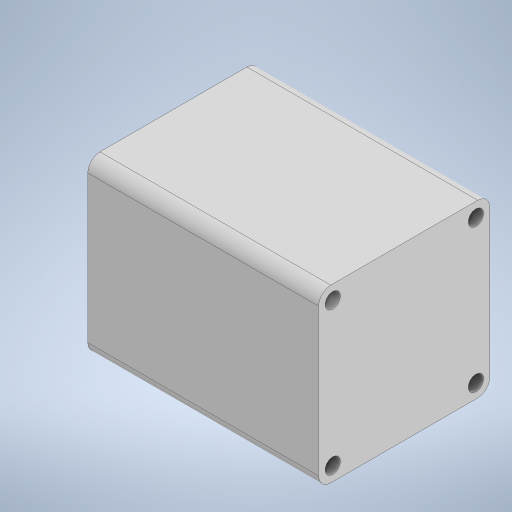
# Autodesk Inventor part: Nema23
Saved by Autodesk Inventor 2023 (Build 270158000, 158)
## iProperties
Created: 2022-04-29
Part Number: Nema23
Material: Generic
Document SubType Name: Modeling
Designer: plebbb
Density: 4.42433 g/cm^3
Appearance: Default
Mass: 1050 g
Surface Area: 282.466 cm^2
Volume: 237.324 cm^3
Author: plebbb
Autodesk Inventor part; units mm, degrees
ref_plane "YZ Plane" through (0, 0, 0) normal (1, 0, 0) x (0, 1, 0)
ref_plane "XZ Plane" through (0, 0, 0) normal (0, 1, 0) x (-1, 0, 0)
ref_plane "XY Plane" through (0, 0, 0) normal (0, 0, 1) x (1, 0, 0)
sketch "Sketch1" plane through (0, 0, 0) normal (1, 0, 0) x (0, 1, 0)
  line L0 (52.4, 0) -> (4, 0)
  line L1 (0, -4) -> (0, -52.4)
  line L2 (4, -56.4) -> (52.4, -56.4)
  line L3 (56.4, -52.4) -> (56.4, -4)
  line L4 (51.77, -4.63) -> (4.63, -4.63) construction
  line L5 (4.63, -4.63) -> (4.63, -51.77) construction
  line L6 (4.63, -51.77) -> (51.77, -51.77) construction
  line L7 (51.77, -51.77) -> (51.77, -4.63) construction
  circle A0 centre (51.77, -4.63) radius 2.5
  circle A1 centre (51.77, -51.77) radius 2.5
  circle A2 centre (4.63, -4.63) radius 2.5
  circle A3 centre (4.63, -51.77) radius 2.5
  arc A4 (56.4, -4) -> (52.4, 0) centre (52.4, -4) ccw
  arc A5 (52.4, -56.4) -> (56.4, -52.4) centre (52.4, -52.4) ccw
  arc A6 (0, -52.4) -> (4, -56.4) centre (4, -52.4) ccw
  arc A7 (4, 0) -> (0, -4) centre (4, -4) ccw
  point P0 (0, 0)
  point P1 (56.4, 0)
  point P2 (0, 0)
  point P3 (56.4, -56.4)
  point P4 (56.4, -28.2)
  point P5 (51.77, -28.2)
  point P6 (28.2, -51.77)
  point P7 (28.2, -56.4)
  dimension "d0" = 56.4
  dimension "d1" = 47.14
  dimension "d2" = 5
  dimension "d3" = 4
  dimension "d4" = 4
  dimension "d5" = 4
  dimension "d6" = 4
  constraints: 16 end point, 8 centre point, 8 point on circle, 8 tangent, 6 point on line, 5 coincident, 4 midpoint, 4 parallel, 4 perpendicular, 3 equal radius, 2 horizontal, 1 horizontal alignment, 1 vertical alignment
  measures "d0" distance of point (56.4, -56.4) point (56.4, 0)
  measures "d1" distance of L6.end L4.start
  measures "d2" diameter of A0
  measures "d3" radius of A4
  measures "d4" radius of A5
  measures "d5" radius of A6
  measures "d6" radius of A7
extrude "Extrusion1" add sketch "Sketch1" along normal blind 76
sketch "Sketch2" plane through (0, 0, 0) normal (-1, 0, 0) x (0, 0, 1)
  circle A0 centre (-28.2, 28.2) radius 19.05
  line L0 (-52.4, 56.4) -> (-4, 56.4) projected
  line L1 (-56.4, 4) -> (-56.4, 52.4) projected
  point P0 (0, 0)
  point P1 (-28.2, 56.4)
  point P2 (-56.4, 28.2)
  dimension "d9" = 38.1
  constraints: 2 midpoint, 1 centre point, 1 horizontal alignment, 1 vertical alignment
  measures "d9" diameter of A0
extrude "Extrusion2" add sketch "Sketch2" along normal blind 1.6
sketch "Sketch3" plane through (-1.6, 28.2, -28.2) normal (-1, 0, 0) x (0, 0, 1)
  circle A0 centre (0, 0) radius 4
  circle A1 centre (0, 0) radius 19.05 construction
  point P0 (28.2, -28.2)
  dimension "d12" = 8
  constraints: 1 centre point, 1 concentric
  measures "d12" diameter of A0
extrude "Extrusion3" add sketch "Sketch3" along normal blind 20
body "Solid1"
